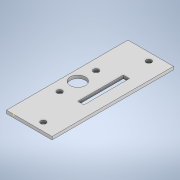
# Autodesk Inventor part: Sensoren plaat
Saved by Autodesk Inventor 2022 (Build 260153000, 153)
## iProperties
Created: 2022-10-10
Part Number: Sensoren plaat
Material: Generic
Document SubType Name: Modeling
Designer: Kilian De Ruyck
Density: 1 g/cm^3
Appearance: Default
Author: Kilian De Ruyck
Autodesk Inventor part; units mm, degrees
ref_plane "YZ Plane" through (0, 0, 0) normal (1, 0, 0) x (0, 1, 0)
ref_plane "XZ Plane" through (0, 0, 0) normal (0, 1, 0) x (-1, 0, 0)
ref_plane "XY Plane" through (0, 0, 0) normal (0, 0, 1) x (1, 0, 0)
sketch "Sketch21" plane through (0, 0, 0) normal (0, 1, 0) x (-1, 0, 0)
  line L0 (0, 0) -> (-25, 0)
  line L1 (-25, 0) -> (-25, -80)
  line L2 (-25, -80) -> (0, -80)
  line L3 (0, -80) -> (0, 0)
  dimension "d227" = 25
  dimension "d228" = 80
  constraints: 8 end point, 2 parallel, 1 horizontal, 1 perpendicular
  measures "d227" distance of L2.end L1.end
  measures "d228" distance of L2.end L0.start
extrude "Extrusion13" add sketch "Sketch21" along normal blind 2
sketch "Sketch22" plane through (0, 2, 0) normal (0, 1, 0) x (1, 0, 0)
  line L0 (0, 80) -> (0, 0) projected
  line L1 (0, 0) -> (25, 0) projected
  point P0 (14, 5.263)
  point P1 (14, 74.737)
  dimension "d231" = 14
  dimension "d232" = 14
  dimension "d233" = 69.474
  dimension "d234" = 5.263
  measures "d231" distance from line of L0 point (14, 5.263)
  measures "d232" distance from line of L0 point (14, 74.737)
  measures "d233" distance of point (14, 74.737) point (14, 5.263)
  measures "d234" distance from line of L1 point (14, 5.263)
hole "Hole7" at (14, 2, -5.263) at (14, 2, -74.737) direction (0, -1, 0) diameter 3.5 depth 2
sketch "Sketch23" plane through (0, 2, 0) normal (0, 1, 0) x (1, 0, 0)
  point P0 (0, 0)
sketch "Sketch24" plane through (0, 2, 0) normal (0, 1, 0) x (1, 0, 0)
  line L0 (13.482, 28.465) -> (17.482, 28.465)
  line L1 (17.482, 28.465) -> (17.482, 58.465)
  line L2 (17.482, 58.465) -> (13.482, 58.465)
  line L3 (13.482, 58.465) -> (13.482, 28.465)
  circle A0 centre (14, 5.263) radius 1.75 projected
  line L4 (0, 80) -> (0, 0) projected
  dimension "d242" = 4
  dimension "d243" = 30
  dimension "d244" = 23.202
  dimension "d245" = 13.482
  constraints: 8 end point, 2 parallel, 1 horizontal, 1 perpendicular
  measures "d242" distance of L2.end L1.end
  measures "d243" distance of L1.end L0.end
  measures "d244" distance from line of A0.centre L0
  measures "d245" distance between parallel lines of L4 L3
extrude "Extrusion14" cut sketch "Sketch24" against normal blind 10 contours L3 L2 L1 L0
sketch "Sketch26" plane through (0, 2, 0) normal (0, 1, 0) x (1, 0, 0)
  line L0 (25, 0) -> (25, 80) projected
  line L1 (0, 0) -> (25, 0) projected
  point P0 (2, 40)
  dimension "d257" = 23
  dimension "d258" = 40
  measures "d257" distance from line of L0 point (2, 40)
  measures "d258" distance from line of L1 point (2, 40)
hole "Hole9" at (2, 2, -40) direction (0, -1, 0) diameter 10 depth 2
sketch "Sketch27" plane through (0, 2, 0) normal (0, 1, 0) x (1, 0, 0)
  arc A0 (0, 35.4174) -> (0, 44.5826) centre (2, 40) ccw projected
  point P0 (0, 0)
  point P1 (2, 28)
  point P2 (2, 52)
  dimension "d266" = 12
  dimension "d267" = 12
  dimension "d268" = 0
  dimension "d269" = 0
  measures "d266" distance of A0.centre point (2, 52)
  measures "d267" distance of A0.centre point (2, 28)
  measures "d268" horizontal distance of A0.centre point (2, 52)
  measures "d269" horizontal distance of point (2, 28) A0.centre
hole "Hole10" at (2, 2, -28) at (2, 2, -52) direction (0, -1, 0) diameter 3.5 depth 2
sketch "Sketch28" plane through (0, 2, 0) normal (0, 1, 0) x (1, 0, 0)
  line L0 (0, 0) -> (25, 0) projected
  line L1 (0, 0) -> (-5, 0)
  line L2 (-5, 0) -> (-5, 80)
  line L3 (-5, 80) -> (0, 80)
  line L4 (0, 80) -> (0, 0)
  dimension "d277" = 5
  dimension "d278" = 80
  constraints: 8 end point, 2 parallel, 1 horizontal, 1 perpendicular
  measures "d277" distance of L2.end L3.end
  measures "d278" distance of L1.end L2.end
extrude "Extrusion15" add sketch "Sketch28" against normal blind 2
sketch "Sketch29" plane through (0, 2, 0) normal (0, 1, 0) x (1, 0, 0)
  arc A0 (0, 35.4174) -> (0, 44.5826) centre (2, 40) ccw projected
  circle A1 centre (2, 40) radius 5
  point P0 (0, 0)
  point P1 (0, 44.5826)
  point P2 (0, 35.4174)
  constraints: 1 centre point, 1 coincident
extrude "Extrusion16" cut sketch "Sketch29" against normal blind 2
equation "\"d232\" = d231"
equation "\"d267\" = d266"
body "Solid2"
